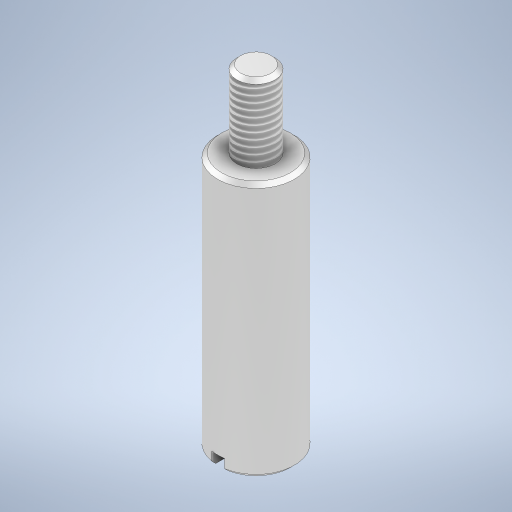
# Autodesk Inventor part: BRU-320S
Saved by Autodesk Inventor 2024.2 (Build 282272000, 272)
## iProperties
Created: 2024-01-03
Part Number: BRU-320S
Material: Stainless Steel AISI 304
Document SubType Name: Modeling
Designer: Masato Kubotera
Density: 8 g/cm^3
Appearance: Chrome - Satin
Catalog Web Link: https://www.hirosugi-net.co.jp/shop/g/g8785/
Vendor: HIROSUGI
Mass: 2.1006 g
Surface Area: 3.22831 cm^2
Volume: 0.262575 cm^3
Author: Masato Kubotera
Autodesk Inventor part; units mm, degrees
ref_plane "YZ Plane" through (0, 0, 0) normal (1, 0, 0) x (0, 1, 0)
ref_plane "XZ Plane" through (0, 0, 0) normal (0, 1, 0) x (-1, 0, 0)
ref_plane "XY Plane" through (0, 0, 0) normal (0, 0, 1) x (1, 0, 0)
sketch "Sketch1" plane through (0, 0, 0) normal (0, 1, 0) x (-1, 0, 0)
  line L0 (0, 0) -> (-3, 0)
  line L1 (-3, 0) -> (-3, 20)
  line L2 (-3, 20) -> (-1.5, 20)
  line L3 (-1.5, 20) -> (-1.5, 26)
  line L4 (-1.5, 26) -> (0, 26)
  line L5 (0, 26) -> (0, 0)
  dimension "d1" = 6
  dimension "d2" = 20
  dimension "d3" = 3
  dimension "d4" = 6
  constraints: 12 end point, 3 horizontal, 2 vertical, 1 perpendicular
  measures "d1" distance of L2.end L3.end
  measures "d2" distance of L0.end L1.end
  measures "d3" diameter of L3 L5
  measures "d4" diameter of L1 L5
revolve "Revolution1" add sketch "Sketch1" angle 360 about axis through (0, 0, 26) along (0, 0, -1)
sketch "Sketch2" plane through (0, 0, 0) normal (0, 0, -1) x (-1, 0, 0)
  line L0 (-3, -0.5) -> (3, -0.5)
  line L1 (3, -0.5) -> (3, 0.5)
  line L2 (3, 0.5) -> (-3, 0.5)
  line L3 (-3, 0.5) -> (-3, -0.5)
  line L4 (-3, -0.5) -> (3, 0.5) construction
  line L5 (3, -0.5) -> (-3, 0.5) construction
  circle A0 centre (0, 0) radius 3 projected
  dimension "d6" = 1
  constraints: 12 end point, 2 midpoint, 2 parallel, 1 horizontal, 1 perpendicular, 1 tangent
  measures "d6" distance of L1.end L0.end
extrude "Extrusion1" cut sketch "Sketch2" against normal blind 1 contours L3 A0 L0 | A0 L2 L0 | L3 L2 A0 | A0 L1 L0 | A0 L2 L1
hole "Hole1" at (0, 0, 0) direction (0, 0, 1) diameter 2.459 depth 6 thread size "M3x0.5" class "6H" standard "ANSI Metric M Profile"
thread "Thread1" size "M3x0.5" class "6g" standard "ANSI Metric M Profile" full length
chamfer "Chamfer1" distance 0.3 angle 45 7 edges at (-3, 0, 20) (0, 3, 0) (0, -3, 0) (0, -1.2295, 0) (-0.6697, 1.0311, 0) (0.6697, 1.0311, 0) (-1.5, 0, 26)
body "Solid1"
